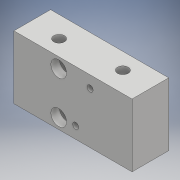
# Autodesk Inventor part: KOGANEI_BDA10X15
Saved by Autodesk Inventor 2018 (Build 220112000, 112)
## iProperties
Created: 2018-04-23
Part Number: KOGANEI_BDA10X15
Material: 一般
Document SubType Name: Modeling
Designer: Take
Density: 1 g/cm^3
Appearance: 既定
Author: Take
Autodesk Inventor part; units mm, degrees
ref_plane "YZ Plane" through (0, 0, 0) normal (1, 0, 0) x (0, 1, 0)
ref_plane "XZ Plane" through (0, 0, 0) normal (0, 1, 0) x (-1, 0, 0)
ref_plane "XY Plane" through (0, 0, 0) normal (0, 0, 1) x (1, 0, 0)
sketch "スケッチ1" plane through (0, 0, 0) normal (0, 1, 0) x (-1, 0, 0)
  line L0 (0, 0) -> (45.1, 0)
  line L1 (45.1, 0) -> (45.1, -24.1)
  line L2 (45.1, -24.1) -> (0, -24.1)
  line L3 (0, -24.1) -> (0, 0)
  dimension "d0" = 45.1
  dimension "d1" = 24.1
  constraints: 8 end point, 2 parallel, 1 horizontal, 1 perpendicular
  measures "d0" distance of L1.end L2.end
  measures "d1" distance of L0.end L1.end
extrude "押し出し1" add sketch "スケッチ1" along normal blind 14
sketch "スケッチ2" plane through (0, 14, 0) normal (0, 1, 0) x (1, 0, 0)
  line L0 (-45.1, 0) -> (0, 0) projected
  line L1 (-28, 0) -> (-28, 24.1)
  line L2 (0, 24.1) -> (-45.1, 24.1) projected
  point P0 (-28, 4)
  point P1 (-28, 20.1)
  dimension "d4" = 4
  dimension "d5" = 4
  constraints: 4 point on line, 2 end point, 1 vertical
  measures "d4" distance from line of point (-28, 4) L0
  measures "d5" distance from line of L2 point (-28, 20.1)
hole "穴1" at (-28, 14, -4) at (-28, 14, -20.1) direction (0, -1, 0) diameter 3 end through all counterbore diameter 6 counterbore depth 3.3
sketch "スケッチ3" plane through (0, 0, 0) normal (0, -1, 0) x (1, 0, 0)
  circle A0 centre (-28, -20.1) radius 1.5 projected
  line L0 (-28, -20.1) -> (-28, 0)
  circle A1 centre (-28, -20.1) radius 3 projected
  circle A2 centre (-28, -4) radius 1.5 projected
  point P0 (0, 0)
  constraints: 2 coincident, 2 end point, 1 vertical
hole "穴2" at (-28, 0, -20.1) at (-28, 0, -4) direction (0, 1, 0) diameter 3 end through all counterbore diameter 6 counterbore depth 3.3
sketch "スケッチ4" plane through (0, 0, 0) normal (0, -1, 0) x (1, 0, 0)
  line L0 (0, 0) -> (-45.1, 0) projected
  line L1 (-16, 0) -> (-16, -23.8904)
  line L2 (0, -24.1) -> (-45.1, -24.1) projected
  line L3 (-21.5, -24.1) -> (-21.5, 0)
  point P0 (-16, -4.5)
  point P1 (-21.5, -19.6)
  dimension "d20" = 4.5
  dimension "d21" = 4.5
  constraints: 5 point on line, 4 end point, 1 perpendicular, 1 vertical
  measures "d20" distance from line of L0 point (-16, -4.5)
  measures "d21" distance from line of point (-21.5, -19.6) L2
hole "穴3" at (-16, 0, -4.5) at (-21.5, 0, -19.6) direction (0, 1, 0) diameter 2.3 end through all
sketch "スケッチ5" plane through (-45.1, 0, -24.1) normal (-1, 0, 0) x (0, 0, 1)
  line L0 (0, 14) -> (24.1, 14) projected
  line L1 (12.05, 14) -> (12.05, 0)
  circle A0 centre (12.05, 7) radius 3.05
  circle A1 centre (12.05, 7) radius 2.5
  point P0 (24.1, 0)
  dimension "d40" = 6.1
  dimension "d41" = 5
  constraints: 2 centre point, 2 coincident, 2 end point, 2 midpoint, 1 vertical
  measures "d40" diameter of A0
  measures "d41" diameter of A1
sketch "スケッチ6" plane through (-45.1, 0, 0) normal (0, 0, 1) x (1, 0, 0)
  line L0 (11.25, 13.7757) -> (11.25, 0)
  line L1 (0, 0) -> (0, 14) projected
  line L2 (45.1, 0) -> (0, 0) projected
  line L3 (45.1, 14) -> (0, 14) projected
  line L4 (33.85, 14) -> (33.85, 0)
  line L5 (45.1, 0) -> (45.1, 14) projected
  point P0 (11.25, 6)
  point P1 (33.85, 7.75)
  dimension "d29" = 11.25
  dimension "d30" = 6
  dimension "d31" = 11.25
  dimension "d32" = 6.25
  constraints: 4 end point, 4 point on line, 1 perpendicular, 1 vertical
  measures "d29" distance between parallel lines of L0 L1
  measures "d30" distance from line of point (11.25, 6) L2
  measures "d31" distance between parallel lines of L4 L5
  measures "d32" distance from line of L3 point (33.85, 7.75)
hole "穴4" at (-11.25, 7.75, 0) at (-33.85, 6, 0) direction (0, 0, -1) diameter 4.1 depth 5.8 tip angle 118
extrude "押し出し2" add sketch "スケッチ5" along normal blind 1 contours A0 L1 A1 | L1 A1 A0
sketch "スケッチ8" plane through (-45.1, 0, -24.1) normal (-1, 0, 0) x (0, 0, 1)
  circle A0 centre (12.05, 7) radius 3.05 projected
  point P0 (24.1, 0)
  constraints: 2 coincident
hole "穴5" at (-45.1, 7, -12.05) direction (1, 0, 0) diameter 5 depth 20
